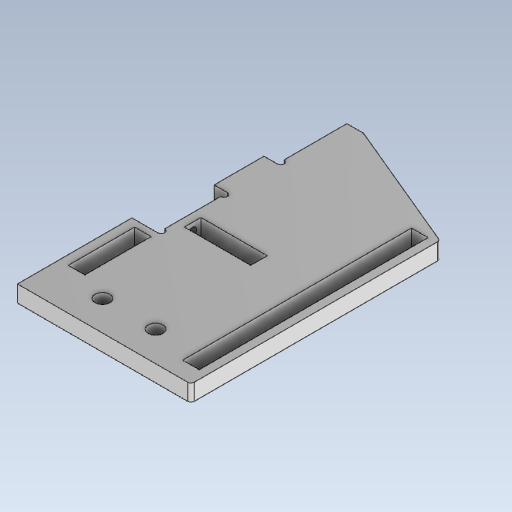
# Autodesk Inventor part: Trunk_lower_flank_frame
Saved by Autodesk Inventor 2020.4 (Build 244396000, 396)
## iProperties
Created: 2021-09-11
Part Number: Trunk_lower_flank_frame
Material: アルミニウム 2014-T4
Document SubType Name: Modeling
Designer: Masato Kubotera
Density: 2.8 g/cm^3
Appearance: 滑らか - 淡い灰色
Mass: 27.0746 g
Surface Area: 75.3869 cm^2
Volume: 9.66951 cm^3
Description: A2017 T5
Author: Masato Kubotera
Autodesk Inventor part; units mm, degrees
ref_plane "YZ Plane" through (0, 0, 0) normal (1, 0, 0) x (0, 1, 0)
ref_plane "XZ Plane" through (0, 0, 0) normal (0, 1, 0) x (-1, 0, 0)
ref_plane "XY Plane" through (0, 0, 0) normal (0, 0, 1) x (1, 0, 0)
derived "Trunk_vertical_frame_03.ipt"
sketch "スケッチ1" plane through (0, 0, 0) normal (0, 0, 1) x (1, 0, 0)
  circle A0 centre (0, 0) radius 11 projected
  line L0 (-0.3073, 13.5) -> (26.6927, 13.5) construction
  line L1 (26.6927, 13.5) -> (26.6927, -13.5) construction
  line L2 (26.6927, -13.5) -> (-0.3073, -13.5) construction
  line L3 (-0.3073, -13.5) -> (-0.3073, 13.5) construction
  line L4 (-0.3073, 13.5) -> (26.6927, -13.5) construction
  line L5 (26.6927, 13.5) -> (-0.3073, -13.5) construction
  line L6 (-12, 16) -> (39.5, 16) construction
  line L7 (39.5, 16) -> (39.5, -16) construction
  line L8 (39.5, -16) -> (-12, -16) construction
  line L9 (-12, -16) -> (-12, 16) construction
  line L10 (-12, 16) -> (39.5, -16) construction
  line L11 (39.5, 16) -> (-12, -16) construction
  circle A1 centre (-0.3073, 13.5) radius 1.35 projected
  arc A2 (0, 16) -> (-12, 10.583) centre (0, 0) ccw construction
  line L12 (-12, 0) -> (39.5, 0) projected
  circle A3 centre (26.6927, 13.5) radius 1.35 projected
  arc A4 (-12, -10.583) -> (0, -16) centre (0, 0) ccw construction
  circle A5 centre (26.6927, -13.5) radius 1.35 projected
  circle A6 centre (-0.3073, -13.5) radius 1.35 projected
  arc A7 (0, 16.05) -> (-12.05, 10.6019) centre (0, 0) ccw projected
  line L13 (0, 16.05) -> (39.55, 16.05) projected
  line L14 (39.55, 16.05) -> (39.55, 13.3) projected
  line L15 (-12.05, 10.6019) -> (-12.05, 0) projected
  arc A8 (-11.5146, 11.1811) -> (-12.05, 9.86) centre (-11.0677, 10.2309) ccw projected
  line L16 (-12.05, 10.6019) -> (-11.0677, 10.2309) construction
  arc A9 (39.55, 14.5651) -> (38.0651, 16.05) centre (38.8075, 15.3075) ccw projected
  line L17 (38.8075, 15.3075) -> (39.55, 16.05) construction
  arc A10 (38.0651, -16.05) -> (39.55, -14.5651) centre (38.8075, -15.3075) ccw projected
  line L18 (-12.05, -10.6019) -> (-12.05, 0) projected
  arc A11 (-12.05, -9.86) -> (-11.5146, -11.1811) centre (-11.0677, -10.2309) ccw projected
  arc A12 (-12.05, -10.6019) -> (0, -16.05) centre (0, 0) ccw projected
  line L19 (0, -16.05) -> (39.55, -16.05) projected
  line L20 (39.55, 13.3) -> (42.05, 13.3) projected
  line L21 (42.05, 13.3) -> (42.05, -1.8) projected
  line L22 (42.05, -1.8) -> (39.55, -1.8) projected
  line L23 (39.55, -1.8) -> (39.55, -14.5651) projected
  line L24 (39.5, 13.25) -> (42, 13.25) construction
  line L25 (42, 13.25) -> (42, -1.75) construction
  line L26 (42, -1.75) -> (39.5, -1.75) construction
  line L27 (42, 5.75) -> (39.5, 5.75) construction
  arc A13 (42.05, 11.8151) -> (40.5651, 13.3) centre (41.3075, 12.5575) ccw projected
  line L28 (41.3075, 12.5575) -> (42.05, 13.3) construction
  arc A14 (40.5651, -1.8) -> (42.05, -0.3151) centre (41.3075, -1.0575) ccw projected
  circle A15 centre (-15.5, 19) radius 1.6 projected
  line L29 (-18, 22) -> (-13, 22) construction
  line L30 (-13, 22) -> (-13, -10.5) construction
  line L31 (-13, -10.5) -> (-18, -10.5) construction
  line L32 (-18, -10.5) -> (-18, 22) construction
  line L33 (-18, 22) -> (-13, -10.5) construction
  line L34 (-13, 22) -> (-18, -10.5) construction
  line L35 (-18, 5.75) -> (-13, 5.75) construction
  line L36 (-15.5, 22) -> (-15.5, -10.5) construction
  line L37 (-18, 13.25) -> (-15.5, 13.25) construction
  line L38 (-15.5, 13.25) -> (-15.5, -1.75) construction
  line L39 (-15.5, -1.75) -> (-18, -1.75) construction
  line L40 (-18, 13.25) -> (-15.5, -1.75) construction
  line L41 (-15.5, 13.25) -> (-18, -1.75) construction
  line L42 (-15.45, -1.8) -> (-18.05, -1.8) projected
  line L43 (-18.05, -1.8) -> (-18.05, 13.3) projected
  line L44 (-18.05, 13.3) -> (-15.45, 13.3) projected
  line L45 (-15.45, 13.3) -> (-15.45, -1.8) projected
  line L46 (-15.45, -1.8) -> (-18.05, 13.3) construction
  line L47 (-18.05, -1.8) -> (-15.45, 13.3) construction
  line L48 (-16.75, 13.3) -> (-16.75, -1.8) construction
  arc A16 (-18.05, 13.3) -> (-18.05, 11.2) centre (-18.05, 12.25) ccw projected
  arc A17 (-15.45, 11.2) -> (-15.45, 13.3) centre (-15.45, 12.25) ccw projected
  arc A18 (-18.05, 0.3) -> (-18.05, -1.8) centre (-18.05, -0.75) ccw projected
  arc A19 (-15.45, -1.8) -> (-15.45, 0.3) centre (-15.45, -0.75) ccw projected
  circle A20 centre (-15.5, -7.5) radius 1.6 projected
  line L49 (13.1927, 16) -> (13.1927, -16) construction
  circle A21 centre (42, 19) radius 1.6 projected
  line L50 (39.5, 22) -> (44.5, 22) construction
  line L51 (44.5, 22) -> (44.5, -10.5) construction
  line L52 (44.5, -10.5) -> (39.5, -10.5) construction
  line L53 (39.5, 22) -> (44.5, -10.5) construction
  line L54 (44.5, 22) -> (39.5, -10.5) construction
  line L55 (42, 22) -> (42, -10.5) construction
  circle A22 centre (42, -7.5) radius 1.6 projected
  line L56 (-12, 23.25) -> (-12, 18.25) construction
  line L57 (-18, 24.5) -> (44.5, 24.5) projected
  line L58 (-18, 24.5) -> (-23, 22) projected
  line L59 (44.5, 24.5) -> (47.5, 22) projected
  line L60 (-23, 22) -> (-23, -10.75) projected
  line L61 (47.5, 22) -> (47.5, -18.25) projected
  line L62 (47.5, -18.25) -> (76.5, -33.25) projected
  line L63 (-23, -10.75) -> (-33.5, -16) projected
  line L64 (-33.5, -16) -> (-33.5, -96.5) projected
  line L65 (76.5, -33.25) -> (76.5, -93.8101) projected
  line L66 (76.5, -93.8101) -> (23, -104.5) construction
  line L67 (23, -104.5) -> (-17, -104.5) construction
  line L68 (-17, -104.5) -> (-33.5, -96.5) construction
  circle A23 centre (-12, -99.5) radius 1.6 construction
  circle A24 centre (3, -99.5) radius 1.6 construction
  line L69 (-17, -104.5) -> (-17, -94.5) construction
  line L70 (-17, -94.5) -> (23, -94.5) construction
  line L71 (23, -94.5) -> (23, -104.5) construction
  line L72 (-17, -99.5) -> (23, -99.5) construction
  line L73 (3, -94.5) -> (3, -104.5) construction
  circle A25 centre (18, -99.5) radius 1.6 construction
  circle A26 centre (-13.5, -61.75) radius 1.6 projected
  line L74 (-23.5, -65.75) -> (66.5, -65.75) projected
  line L75 (66.5, -65.75) -> (66.5, -84.5) projected
  line L76 (66.5, -84.5) -> (-23.5, -84.5) projected
  line L77 (-23.5, -84.5) -> (-23.5, -65.75) projected
  line L78 (-23.5, -33.25) -> (66.5, -33.25) projected
  line L79 (66.5, -33.25) -> (66.5, -57.75) projected
  line L80 (66.5, -57.75) -> (-23.5, -57.75) projected
  line L81 (-23.5, -57.75) -> (-23.5, -33.25) projected
  circle A27 centre (-13.5, -61.75) radius 4 construction
  arc A28 (-11.4334, -102.3) -> (-9.8584, -101.3907) centre (-10.9084, -101.3907) ccw construction
  line L82 (-9.2918, -100.4093) -> (-9.8584, -101.3907) construction
  arc A29 (-9.2918, -100.4093) -> (-9.2918, -98.5907) centre (-9.8168, -99.5) ccw construction
  line L83 (-9.8584, -97.6093) -> (-9.2918, -98.5907) construction
  arc A30 (-9.8584, -97.6093) -> (-11.4334, -96.7) centre (-10.9084, -97.6093) ccw construction
  line L84 (-12.5666, -96.7) -> (-11.4334, -96.7) construction
  arc A31 (-12.5666, -96.7) -> (-14.1416, -97.6093) centre (-13.0916, -97.6093) ccw construction
  line L85 (-14.7082, -98.5907) -> (-14.1416, -97.6093) construction
  arc A32 (-14.7082, -98.5907) -> (-14.7082, -100.4093) centre (-14.1832, -99.5) ccw construction
  line L86 (-14.1416, -101.3907) -> (-14.7082, -100.4093) construction
  arc A33 (-14.1416, -101.3907) -> (-12.5666, -102.3) centre (-13.0916, -101.3907) ccw construction
  line L87 (-11.4334, -102.3) -> (-12.5666, -102.3) construction
  arc A34 (5.7082, -100.4093) -> (5.7082, -98.5907) centre (5.1832, -99.5) ccw construction
  line L88 (5.1416, -97.6093) -> (5.7082, -98.5907) construction
  line L89 (5.7082, -100.4093) -> (5.1416, -101.3907) construction
  arc A35 (3.5666, -102.3) -> (5.1416, -101.3907) centre (4.0916, -101.3907) ccw construction
  arc A36 (5.1416, -97.6093) -> (3.5666, -96.7) centre (4.0916, -97.6093) ccw construction
  line L90 (2.4334, -96.7) -> (3.5666, -96.7) construction
  arc A37 (2.4334, -96.7) -> (0.8584, -97.6093) centre (1.9084, -97.6093) ccw construction
  line L91 (0.2918, -98.5907) -> (0.8584, -97.6093) construction
  arc A38 (0.2918, -98.5907) -> (0.2918, -100.4093) centre (0.8168, -99.5) ccw construction
  line L92 (0.8584, -101.3907) -> (0.2918, -100.4093) construction
  arc A39 (0.8584, -101.3907) -> (2.4334, -102.3) centre (1.9084, -101.3907) ccw construction
  line L93 (3.5666, -102.3) -> (2.4334, -102.3) construction
  arc A40 (20.7082, -100.4093) -> (20.7082, -98.5907) centre (20.1832, -99.5) ccw construction
  line L94 (20.1416, -97.6093) -> (20.7082, -98.5907) construction
  line L95 (20.7082, -100.4093) -> (20.1416, -101.3907) construction
  arc A41 (18.5666, -102.3) -> (20.1416, -101.3907) centre (19.0916, -101.3907) ccw construction
  arc A42 (20.1416, -97.6093) -> (18.5666, -96.7) centre (19.0916, -97.6093) ccw construction
  line L96 (17.4334, -96.7) -> (18.5666, -96.7) construction
  arc A43 (17.4334, -96.7) -> (15.8584, -97.6093) centre (16.9084, -97.6093) ccw construction
  line L97 (15.2918, -98.5907) -> (15.8584, -97.6093) construction
  arc A44 (15.2918, -98.5907) -> (15.2918, -100.4093) centre (15.8168, -99.5) ccw construction
  line L98 (15.8584, -101.3907) -> (15.2918, -100.4093) construction
  arc A45 (15.8584, -101.3907) -> (17.4334, -102.3) centre (16.9084, -101.3907) ccw construction
  line L99 (18.5666, -102.3) -> (17.4334, -102.3) construction
  line L100 (-33.5, -94.5) -> (58, -94.5)
  line L101 (58, -94.5) -> (58, -143)
  line L102 (-33.5, -139) -> (23.51, -139)
  arc A46 (-12.5, -139) -> (-14.6, -139) centre (-13.55, -139) ccw
  line L103 (-12.5, -139) -> (-12.5, -143)
  line L104 (2.5, -143) -> (2.5, -139)
  arc A47 (4.6, -139) -> (2.5, -139) centre (3.55, -139) ccw
  line L105 (-30.5, -139) -> (-30.5, -143) construction
  line L106 (-33.5, -139) -> (-33.5, -143) construction
  line L107 (23.5, -139) -> (23.5, -143) construction
  line L108 (20.5, -139) -> (20.5, -143) construction
  line L109 (-33.5, -143) -> (2.5, -143) construction
  line L110 (2.5, -143) -> (58, -143) construction
  line L111 (23.51, -139) -> (58, -139) construction
  arc A48 (23.51, -139) -> (21.41, -139) centre (22.46, -139) ccw
  line L112 (55.0096, -101.3327) -> (55.0096, -143.0216)
  line L113 (39.4579, -122.1772) -> (55.0096, -122.1772) construction
  circle A49 centre (49.0096, -114.1772) radius 6 construction
  line L114 (49.0096, -114.1772) -> (49.0096, -122.1772) construction
  circle A50 centre (49.0096, -114.1772) radius 2.25
  line L115 (49.0096, -117.3642) -> (46.2496, -115.7707) construction
  line L116 (46.2496, -115.7707) -> (46.2496, -112.5837) construction
  line L117 (46.2496, -112.5837) -> (49.0096, -110.9902) construction
  line L118 (49.0096, -110.9902) -> (51.7696, -112.5837) construction
  line L119 (51.7696, -112.5837) -> (51.7696, -115.7707) construction
  line L120 (51.7696, -115.7707) -> (49.0096, -117.3642) construction
  arc A51 (48.1003, -116.8392) -> (49.9189, -116.8392) centre (49.0096, -116.3142) ccw
  arc A52 (50.8603, -116.2957) -> (51.7696, -114.7207) centre (50.8603, -115.2457) ccw construction
  arc A53 (51.7696, -113.6337) -> (50.8603, -112.0587) centre (50.8603, -113.1087) ccw construction
  arc A54 (49.9189, -111.5152) -> (48.1003, -111.5152) centre (49.0096, -112.0402) ccw construction
  arc A55 (47.1589, -112.0587) -> (46.2496, -113.6337) centre (47.1589, -113.1087) ccw construction
  arc A56 (46.2496, -114.7207) -> (47.1589, -116.2957) centre (47.1589, -115.2457) ccw construction
  circle A57 centre (49.0096, -130.1772) radius 2.25
  line L121 (49.0096, -126.9902) -> (46.2496, -128.5837) construction
  line L122 (46.2496, -128.5837) -> (46.2496, -131.7707) construction
  line L123 (46.2496, -131.7707) -> (49.0096, -133.3642) construction
  line L124 (49.0096, -133.3642) -> (51.7696, -131.7707) construction
  line L125 (51.7696, -131.7707) -> (51.7696, -128.5837) construction
  line L126 (51.7696, -128.5837) -> (49.0096, -126.9902) construction
  arc A58 (49.9189, -127.5152) -> (48.1003, -127.5152) centre (49.0096, -128.0402) ccw construction
  arc A59 (51.7696, -129.6337) -> (50.8603, -128.0587) centre (50.8603, -129.1087) ccw construction
  arc A60 (50.8603, -132.2957) -> (51.7696, -130.7207) centre (50.8603, -131.2457) ccw construction
  arc A61 (48.1003, -132.8392) -> (49.9189, -132.8392) centre (49.0096, -132.3142) ccw construction
  arc A62 (46.2496, -130.7207) -> (47.1589, -132.2957) centre (47.1589, -131.2457) ccw construction
  arc A63 (47.1589, -128.0587) -> (46.2496, -129.6337) centre (47.1589, -129.1087) ccw construction
  line L127 (-17, -94.5) -> (-33.5, -134)
  line L128 (-21.8485, -134) -> (-33.5, -134) construction
  line L129 (23.51, -146.8041) -> (58, -146.8041)
  line L130 (23.51, -139) -> (23.51, -146.8041)
  line L131 (58, -143) -> (58, -146.8041)
  circle A64 centre (49.0096, -130.1772) radius 6 construction
  circle A65 centre (49.0096, -114.1772) radius 1.55 construction
  circle A66 centre (49.0096, -130.1772) radius 1.55 construction
  line L132 (-12.5, -143) -> (2.5, -143)
  line L133 (-33.5, -134) -> (-33.5, -139)
  line L134 (18, -144) -> (13, -144) construction
  line L135 (13, -144) -> (13, -109) construction
  line L136 (13, -109) -> (18, -109) construction
  line L137 (18, -109) -> (18, -144) construction
  line L138 (18, -144) -> (13, -109) construction
  line L139 (13, -144) -> (18, -109) construction
  line L140 (53, -144) -> (18, -144) construction
  line L141 (18, -144) -> (18, -139) construction
  line L142 (18, -139) -> (53, -139) construction
  line L143 (53, -139) -> (53, -144) construction
  line L144 (53, -144) -> (18, -139) construction
  line L145 (18, -144) -> (53, -139) construction
  line L146 (13, -116.5) -> (18, -116.5)
  line L147 (18, -116.5) -> (18, -136.5)
  line L148 (18, -136.5) -> (13, -136.5)
  line L149 (13, -136.5) -> (13, -116.5)
  line L150 (13, -116.5) -> (18, -136.5) construction
  line L151 (18, -116.5) -> (13, -136.5) construction
  line L152 (45.5, -139) -> (25.5, -139)
  line L153 (25.5, -139) -> (25.5, -144)
  line L154 (25.5, -144) -> (45.5, -144)
  line L155 (45.5, -144) -> (45.5, -139)
  line L156 (45.5, -139) -> (25.5, -144) construction
  line L157 (25.5, -139) -> (45.5, -144) construction
  line L158 (-15.9738, -97) -> (53, -97)
  line L159 (53, -97) -> (53, -102)
  line L160 (53, -102) -> (-15.9738, -102)
  line L161 (-15.9738, -102) -> (-15.9738, -97)
  line L162 (-15.9738, -97) -> (53, -102) construction
  line L163 (53, -97) -> (-15.9738, -102) construction
  point P0 (13.1927, 0)
  point P1 (-15.5, 5.75)
  point P2 (-16.75, 5.75)
  point P3 (13.1927, 0)
  point P4 (42, 5.75)
  point P5 (42, 5.75)
  point P6 (-10.3834, -102.3)
  point P7 (-8.7668, -99.5)
  point P8 (-10.3834, -96.7)
  point P9 (-13.6166, -96.7)
  point P10 (-13.6166, -96.7)
  point P11 (-15.2332, -99.5)
  point P12 (-13.6166, -102.3)
  point P13 (-15.2332, -99.5)
  point P14 (-8.7668, -99.5)
  point P15 (3, -99.5)
  point P16 (6.2332, -99.5)
  point P17 (6.2332, -99.5)
  point P18 (4.6166, -96.7)
  point P19 (4.6166, -102.3)
  point P20 (3, -99.5)
  point P21 (3, -99.5)
  point P22 (1.3834, -96.7)
  point P23 (1.3834, -96.7)
  point P24 (-0.2332, -99.5)
  point P25 (-0.2332, -99.5)
  point P26 (1.3834, -102.3)
  point P27 (18, -99.5)
  point P28 (21.2332, -99.5)
  point P29 (21.2332, -99.5)
  point P30 (19.6166, -96.7)
  point P31 (19.6166, -102.3)
  point P32 (18, -99.5)
  point P33 (18, -99.5)
  point P34 (16.3834, -96.7)
  point P35 (16.3834, -96.7)
  point P36 (14.7668, -99.5)
  point P37 (14.7668, -99.5)
  point P38 (16.3834, -102.3)
  point P39 (51.7696, -115.7707)
  point P40 (51.7696, -112.5837)
  point P41 (49.0096, -110.9902)
  point P42 (46.2496, -112.5837)
  point P43 (46.2496, -115.7707)
  point P44 (51.7696, -128.5837)
  point P45 (51.7696, -131.7707)
  point P46 (49.0096, -133.3642)
  point P47 (46.2496, -131.7707)
  point P48 (46.2496, -128.5837)
  point P49 (-14.1416, -97.6093)
  point P50 (0.8584, -97.6093)
  point P51 (15.8584, -97.6093)
  point P52 (50.8603, -132.2957)
  point P53 (49.9189, -132.8392)
  point P54 (48.1003, -132.8392)
  point P55 (47.1589, -132.2957)
  point P56 (46.2496, -130.7207)
  point P57 (46.2496, -129.6337)
  point P58 (47.1589, -128.0587)
  point P59 (50.8603, -128.0587)
  point P60 (51.7696, -129.6337)
  point P61 (51.7696, -130.7207)
  point P62 (46.2496, -114.7207)
  point P63 (46.2496, -113.6337)
  point P64 (47.1589, -112.0587)
  point P65 (48.1003, -111.5152)
  point P66 (49.9189, -111.5152)
  point P67 (50.8603, -112.0587)
  point P68 (51.7696, -113.6337)
  point P69 (51.7696, -114.7207)
  point P70 (50.8603, -116.2957)
  point P71 (47.1589, -116.2957)
  point P72 (2.5, -139)
  point P73 (2.5, -139)
  point P74 (-0.95, 20.8)
  point P75 (15.95, 20.8)
  point P76 (15.95, 18.2)
  point P77 (15.95, -20.8)
  point P78 (-0.95, -20.8)
  point P79 (15.95, -18.2)
  point P80 (-18.05, 0.3)
  point P81 (-15.45, 0.3)
  point P82 (42.05, -0.3151)
  point P83 (40.5651, -1.8)
  point P84 (-17.9821, -97)
  point P85 (-5, -143)
  point P86 (54.5671, -143)
  point P87 (15.5, -126.5)
  point P88 (35.5, -141.5)
  point P89 (18.5131, -99.5)
  dimension "d2" = 1.05
  dimension "d7" = 1.05
  dimension "d12" = 4
  dimension "d16" = 3
  dimension "d17" = 3
  dimension "d23" = 1.05
  dimension "d34" = 12
  dimension "d36" = 4.5
  dimension "d37" = 5.52
  dimension "d38" = 1.05
  dimension "d41" = 360
  dimension "d43" = 16
  dimension "d47" = 5
  dimension "d75" = 0.01
  dimension "d80" = 3.1
  dimension "d92" = 44.5
  dimension "d93" = 15
  dimension "d94" = 28.5
  dimension "d95" = 28.5
  dimension "d96" = 5
  dimension "d97" = 5
  dimension "d98" = 35
  dimension "d99" = 35
  dimension "d101" = 20
  dimension "d102" = 20
  dimension "d103" = 5
  dimension "d105" = 90
  dimension "d106" = 5
  dimension "d107" = 5
  dimension "d108" = 2.5
  dimension "d109" = 37
  dimension "d110" = 5
  constraints: 126 end point, 34 symmetric about line, 31 point on circle, 21 centre point, 16 perpendicular, 16 point on line, 13 midpoint, 12 parallel, 10 horizontal, 5 coincident, 4 collinear, 3 tangent, 3 vertical, 68 other
  measures "d2" radius of A46
  measures "d7" radius of A47
  measures "d12" distance of L106.start L106.end
  measures "d16" distance of L106.end L105.end
  measures "d17" distance of L107.end L108.end
  measures "d23" radius of A48
  measures "d34" diameter of A49
  measures "d36" diameter of A50
  measures "d37" distance from line of L117 L119.end
  measures "d38" radius of A51
  measures "d43" distance of point (49.01, -130.177) A50.centre
  measures "d47" distance of L127.end L106.start
  measures "d75" distance between parallel lines of L130 L107
  measures "d80" diameter of A65
  measures "d93" distance of L104.start L103.end
  measures "d94" distance of L106.end point (-5, -143)
  measures "d95" horizontal distance of point (-5, -143) L107.start
  measures "d96" distance of L135.end L136.end
  measures "d97" distance of L140.end L141.end
  measures "d98" distance of L140.start L140.end
  measures "d99" distance of L134.end L135.end
  measures "d101" distance of L146.end L147.end
  measures "d102" distance of L153.end L154.end
  measures "d103" distance between parallel lines of L111 L154
  measures "d105" angle of L100 L101
  measures "d106" horizontal distance of L140.start L129.end
  measures "d107" distance of L158.end L159.end
  measures "d108" distance between parallel lines of L158 L100
  measures "d109" distance between parallel lines of L152 L160
  measures "d110" distance from line of L100.end L159
extrude "押し出し1" add sketch "スケッチ1" along normal blind 5 contours L100 L101 L131 L129 L130 A48 L102 A47 A46 L133 L127 | L102 L104 L132 L103
sketch "スケッチ2" plane through (-33.5, -139, 0) normal (0, -1, 0) x (1, 0, 0)
  line L0 (36, 0) -> (36, 5) projected
  line L1 (57.01, 0) -> (57.01, 5) projected
  line L2 (21, 0) -> (21, 5) projected
  point P0 (33.5, 0)
  point P1 (8, 2.5)
  point P2 (0, 0)
  point P3 (49, 2.5)
  dimension "d59" = 2.5
  dimension "d61" = 2.5
  dimension "d86" = 13
  dimension "d87" = 13
  measures "d59" vertical distance of point (0, 0) point (8, 2.5)
  measures "d61" vertical distance of point (0, 0) point (49, 2.5)
  measures "d86" distance from line of point (8, 2.5) L2
  measures "d87" distance from line of point (49, 2.5) L0
hole "穴1" at (-25.5, -139, 2.5) at (15.5, -139, 2.5) direction (0, 1, 0) diameter 2.459 depth 5 thread size "M3x0.5" class "6H" standard "ISO Metric profile"
fillet "フィレット1" radius 1 3 edges at (58, -94.5, 2.5) (-33.5, -134, 2.5) (-17, -94.5, 2.5)
equation "\"d7\" = d2"
equation "\"d23\" = d7"
equation "\"d38\" = d2"
equation "\"d13\" = d10"
equation "\"d10\" = 0.01"
